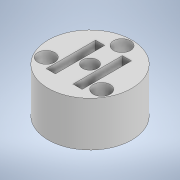
# Autodesk Inventor part: table
Saved by Autodesk Inventor 2020 (Build 240168000, 168)
## iProperties
Created: 2019-06-14
Part Number: table
Material: Generic
Document SubType Name: Modeling
Designer: ColinP
Density: 1 g/cm^3
Appearance: Default
Mass: 13.8064 g
Surface Area: 68.7825 cm^2
Volume: 13.8064 cm^3
Author: ColinP
Autodesk Inventor part; units mm, degrees
ref_plane "YZ Plane" through (0, 0, 0) normal (1, 0, 0) x (0, 1, 0)
ref_plane "XZ Plane" through (0, 0, 0) normal (0, 1, 0) x (-1, 0, 0)
ref_plane "XY Plane" through (0, 0, 0) normal (0, 0, 1) x (1, 0, 0)
sketch "Sketch1" plane through (0, 0, 0) normal (0, 1, 0) x (-1, 0, 0)
  line L0 (0, 0) -> (13.6144, 0)
  circle A0 centre (0, 0) radius 17.78
  dimension "d0" = 13.6144
  dimension "d1" = 35.56
  constraints: 2 coincident, 2 end point, 1 centre point, 1 horizontal
  measures "d0" distance of L0.start L0.end
  measures "d1" diameter of A0
extrude "Extrusion1" add sketch "Sketch1" along normal blind 19.05
sketch "Sketch3" plane through (0, 19.05, 0) normal (0, 1, 0) x (1, 0, 0)
  line L0 (0, 0) -> (0, 13.6144)
  line L1 (0, 0) -> (13.6144, 0) construction
  dimension "d4" = 13.6144
  dimension "d5" = 90
  constraints: 4 end point, 1 horizontal, 1 perpendicular, 1 vertical
  measures "d4" distance of L0.start L0.end
  measures "d5" angle of L1 L0
hole "Hole1" at (0, 19.05, -13.6144) direction (0, -1, 0) diameter 4.9022 end through all counterbore diameter 7.239 counterbore depth 5.08
sketch "Sketch4" plane through (0, 0, 0) normal (0, -1, 0) x (1, 0, 0)
  circle A0 centre (0, -13.6144) radius 2.4511 projected
  line L0 (0, 0) -> (0, -13.6144)
  constraints: 2 end point, 1 vertical
hole "Hole2" at (0, 0, -13.6144) direction (0, 1, 0) diameter 4.9022 depth 6.35
pattern_circular "Circular Pattern1" count 3 over 360 about axis through (0, 0, 0) along (0, 1, 0) of "Hole1", "Hole2"
sketch "Sketch6" plane through (0, 19.05, 0) normal (0, 1, 0) x (1, 0, 0)
  point P0 (0, 0)
  point P1 (0, 0)
  constraints: 1 coincident
hole "Hole3" at (0, 19.05, 0) direction (0, -1, 0) diameter 6.35 end through all
sketch "Sketch13" plane through (0, 0, 0) normal (0, -1, 0) x (1, 0, 0)
  circle A0 centre (11.7904, 6.8072) radius 2.4511 projected
  circle A1 centre (-11.7904, 6.8072) radius 2.4511 projected
  line L0 (11.7904, 6.8072) -> (-11.7904, 6.8072)
  circle A2 centre (0, -13.6144) radius 2.4511 projected
  line L1 (-11.7904, 6.8072) -> (0, -13.6144)
  line L2 (0, -13.6144) -> (11.7904, 6.8072)
  line L3 (0, 6.8072) -> (0, -13.6144)
  line L4 (-11.7904, 6.8072) -> (5.8952, -3.4036)
  line L5 (11.7904, 6.8072) -> (-5.8952, -3.4036)
  circle A3 centre (0, 0) radius 16.0655
  circle A4 centre (5.8952, -3.4036) radius 6.8072
  circle A5 centre (0, 0) radius 17.78 projected
  circle A6 centre (0, 6.8072) radius 6.8072
  circle A7 centre (-5.8952, -3.4036) radius 6.8072
  line L6 (11.7904, 0) -> (5.8952, 3.4036)
  line L7 (0, -6.8072) -> (5.8952, 3.4036)
  line L8 (11.7904, 0) -> (5.8952, -10.2108)
  line L9 (0, -6.8072) -> (5.8952, -10.2108)
  line L10 (5.8952, 3.4036) -> (5.8952, 10.2108)
  line L11 (-5.8952, 10.2108) -> (5.8952, 10.2108)
  line L12 (5.8952, 3.4036) -> (-5.8952, 3.4036)
  line L13 (-5.8952, 10.2108) -> (-5.8952, 3.4036)
  line L14 (-5.8952, 3.4036) -> (0, -6.8072)
  line L15 (-5.8952, -10.2108) -> (0, -6.8072)
  line L16 (-5.8952, 3.4036) -> (-11.7904, 0)
  line L17 (-5.8952, -10.2108) -> (-11.7904, 0)
  line L18 (11.7904, 0) -> (15.0444, 5.6361)
  line L19 (5.8952, -10.2108) -> (2.6412, -15.8469)
  line L20 (5.8952, 10.2108) -> (12.4032, 10.2108)
  line L21 (-5.8952, 10.2108) -> (-12.4032, 10.2108)
  line L22 (-11.7904, 0) -> (-15.0444, 5.6361)
  line L23 (-5.8952, -10.2108) -> (-2.6412, -15.8469)
  line L24 (-12.4032, 10.2108) -> (0, 13.6144)
  line L25 (12.4032, 10.2108) -> (0, 13.6144)
  line L26 (15.0444, 5.6361) -> (11.7904, -6.8072)
  line L27 (2.6412, -15.8469) -> (11.7904, -6.8072)
  line L28 (-2.6412, -15.8469) -> (-11.5062, -7.2578)
  line L29 (-15.0444, 5.6361) -> (-11.5062, -7.2578)
  line L30 (-11.5062, -7.2578) -> (-4.2682, -13.0289)
  line L31 (-4.2682, -13.0289) -> (-6.8619, -14.5263)
  line L32 (-6.8619, -14.5263) -> (-4.2682, -13.0289)
  constraints: 66 end point, 18 point on circle, 8 perpendicular, 4 coincident, 4 midpoint, 3 centre point, 3 point on line, 2 horizontal, 2 tangent, 1 parallel, 1 vertical, 9 other
sketch "Sketch14" plane through (0, 0, 0) normal (0, -1, 0) x (1, 0, 0)
  circle A0 centre (11.7904, 6.8072) radius 2.4511 projected
  circle A1 centre (0, -13.6144) radius 2.4511 projected
  circle A2 centre (-11.7904, 6.8072) radius 2.4511 projected
  point P0 (0, 0)
sketch "Sketch18" plane through (0, 0, 0) normal (0, -1, 0) x (1, 0, 0)
  circle A0 centre (-11.7904, 6.8072) radius 2.4511 projected
  circle A1 centre (-11.7904, 6.8072) radius 4.1697
  circle A2 centre (0, 0) radius 3.7517
  line L0 (-7.6207, 6.8072) -> (-7.6207, -16.064)
  circle A3 centre (0, 0) radius 17.78 projected
  line L1 (-7.6207, 6.8072) -> (-7.6207, 16.064)
  line L2 (-3.7517, 0) -> (-3.7517, -17.4687)
  line L3 (-3.7517, -17.4687) -> (-3.7517, 17.2429)
  circle A4 centre (11.7904, 6.8072) radius 2.4511 projected
  circle A5 centre (11.7904, 6.8072) radius 4.1697
  line L4 (7.6207, 6.8072) -> (7.6207, -16.064)
  line L5 (7.6207, 16.064) -> (7.6207, 6.8072)
  line L6 (-7.6207, 10.9769) -> (-3.7517, 10.9769)
  line L7 (-6.9141, -9.9949) -> (-3.7517, -9.9949)
  line L8 (-7.6207, -9.9949) -> (-6.5754, -9.9949)
  line L9 (3.7517, 10.9769) -> (7.6207, 10.9769)
  line L10 (3.7517, -9.9949) -> (7.6207, -9.9949)
  line L11 (0, 0) -> (3.7517, 0)
  line L12 (3.7517, 0) -> (3.7517, 10.8227)
  line L13 (3.7517, 10.8227) -> (3.7517, -9.9949)
  line L14 (3.7517, 10.8227) -> (3.7517, 10.9769)
  line L15 (7.6207, 10.9769) -> (3.7517, 10.9769)
  point P0 (3.7517, 0)
  constraints: 32 end point, 15 point on line, 6 point on circle, 4 vertical, 3 coincident, 3 collinear, 2 horizontal alignment, 2 perpendicular, 1 centre point, 1 horizontal, 1 parallel, 1 tangent, 4 other
sketch "Sketch17" plane through (0, 0, 0) normal (0, -1, 0) x (1, 0, 0)
  point P0 (0, 0)
extrude "Extrusion6" cut sketch "Sketch18" against normal blind 19.05 contours L1 L6 L3 L2 L7 L8 L0 | L5 L4 L10 L13 L12 L14 L9
sketch "Sketch21" plane through (0, 0, 0) normal (0, -1, 0) x (1, 0, 0)
  circle A0 centre (11.7904, 6.8072) radius 2.4511 projected
  circle A1 centre (0, -13.6144) radius 2.4511 projected
  line L0 (11.7904, 6.8072) -> (0, -13.6144)
  circle A2 centre (-11.7904, 6.8072) radius 2.4511 projected
  line L1 (0, -13.6144) -> (-11.7904, 6.8072)
  line L2 (-11.7904, 6.8072) -> (11.7904, 6.8072)
  line L3 (11.7904, 6.8072) -> (11.7904, -13.6144)
  line L4 (11.7904, -13.6144) -> (0, -13.6144)
  line L5 (0, -13.6144) -> (-11.7904, -13.6144)
  line L6 (-11.7904, -13.6144) -> (-11.7904, 6.8072)
  circle A3 centre (11.7904, -3.4036) radius 0.635
  circle A4 centre (-11.7904, -3.4036) radius 0.635
  point P0 (0, 0)
  dimension "d68" = 1.27
  constraints: 14 end point, 2 centre point, 2 midpoint, 2 point on line, 1 horizontal, 1 perpendicular, 1 vertical
  measures "d68" diameter of A3
hole "Hole6" at (-11.7904, 0, -3.4036) at (11.7904, 0, -3.4036) direction (0, 1, 0) diameter 1.905 depth 6.35
body "Solid1"
